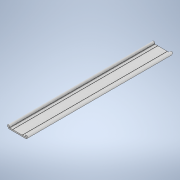
# Autodesk Inventor part: WS_10_80_600
Saved by Autodesk Inventor 2020 (Build 240168000, 168)
## iProperties
Created: 2022-04-07
Part Number: WS_10_80_600
Material: Ogólny
Document SubType Name: Modeling
Designer: mikoma
Density: 1 g/cm^3
Appearance: Domyślna
Author: mikoma
Autodesk Inventor part; units mm, degrees
ref_plane "YZ Plane" through (0, 0, 0) normal (1, 0, 0) x (0, 1, 0)
ref_plane "XZ Plane" through (0, 0, 0) normal (0, 1, 0) x (-1, 0, 0)
ref_plane "XY Plane" through (0, 0, 0) normal (0, 0, 1) x (1, 0, 0)
sketch "Szkic1" plane through (0, 0, 0) normal (0, 0, 1) x (1, 0, 0)
  line L0 (32, 9) -> (42, 9)
  line L1 (37, 14) -> (37, 4)
  line L2 (-20, 5.5) -> (-20, 0)
  line L3 (20, 5.5) -> (20, 0)
  line L4 (20, 5.5) -> (20, 0)
  line L5 (-42.0008, 8.9996) -> (-32, 8.9996)
  line L6 (-37, 14) -> (-37, 4)
  line L7 (-20, 5.5) -> (-20, 0)
  line L8 (12.2798, 0) -> (12.0798, 0.2)
  line L9 (20, 5.2113) -> (19.5, 5.5)
  line L10 (20, 5.2113) -> (20.5, 5.5)
  line L11 (12.2798, 0) -> (28.2798, 0)
  line L12 (20.5, 5.5) -> (31, 5.5)
  line L13 (31, 5.5) -> (32.4315, 6.3265)
  arc A0 (32.4315, 6.3265) -> (32.5486, 6.7229) centre (32.2815, 6.5863) ccw
  line L14 (28.4798, 0.2) -> (36.7798, 0.2)
  arc A1 (37.283, 4.008) -> (37.2798, 3.7085) centre (37.5413, 3.8554) ccw
  line L15 (37.2798, 0.7) -> (37.2798, 3.7085)
  line L16 (36.7798, 0.2) -> (37.2798, 0.7)
  arc A2 (37.283, 4.008) -> (32.5486, 6.7229) centre (37, 9) ccw
  line L17 (28.2798, 0) -> (28.4798, 0.2)
  line L18 (-19.5, 5.5) -> (19.5, 5.5)
  line L19 (-11.7202, 0) -> (-11.5202, 0.2)
  line L20 (-20, 5.2113) -> (-19.5, 5.5)
  line L21 (-20, 5.2113) -> (-20.5, 5.5)
  line L22 (-28, 0) -> (-11.7202, 0)
  line L23 (-28, 0) -> (-28.2, 0.2)
  line L24 (-31, 5.5) -> (-20.5, 5.5)
  line L25 (-31, 5.5) -> (-32.4315, 6.3265)
  arc A3 (-32.5537, 6.7125) -> (-32.4315, 6.3265) centre (-32.2815, 6.5863) ccw
  line L26 (-36.5, 0.2) -> (-28.2, 0.2)
  line L27 (-36.5, 0.2) -> (-37, 0.7)
  line L28 (-37, 0.7) -> (-37, 3.7085)
  arc A4 (-37, 3.7085) -> (-37.2979, 4.008) centre (-37.3, 3.708) ccw
  arc A5 (-32.5537, 6.7125) -> (-37.2979, 4.008) centre (-37.0004, 8.9996) ccw
  line L29 (-11.5202, 0.2) -> (12.0798, 0.2)
  point P0 (0, 0)
  dimension "d0" = 37
  constraints: 60 end point, 18 point on circle, 6 centre point, 6 point on line, 1 horizontal alignment
  measures "d0" horizontal distance of point (0, 0) L27.end
extrude "Wyciągnięcie proste1" add sketch "Szkic1" against normal blind 600
